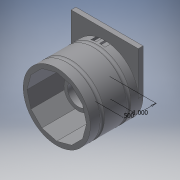
# Autodesk Inventor part: mounting plate
Saved by Autodesk Inventor 2017 (Build 210142000, 142)
## iProperties
Created: 2017-11-23
Part Number: mounting plate
Material: Generic
Document SubType Name: Modeling
Designer: prakh
Density: 1 g/cm^3
Appearance: Default
Author: prakh
Autodesk Inventor part; units mm, degrees
ref_plane "YZ Plane" through (0, 0, 0) normal (1, 0, 0) x (0, 1, 0)
ref_plane "XZ Plane" through (0, 0, 0) normal (0, 1, 0) x (-1, 0, 0)
ref_plane "XY Plane" through (0, 0, 0) normal (0, 0, 1) x (1, 0, 0)
sketch "Sketch1" plane through (0, 0, 0) normal (0, 0, 1) x (1, 0, 0)
  circle A0 centre (0, 0) radius 44.45
  line L0 (-44.45, 44.45) -> (44.45, 44.45)
  line L1 (44.45, 44.45) -> (44.45, -44.45)
  line L2 (44.45, -44.45) -> (-44.45, -44.45)
  line L3 (-44.45, -44.45) -> (-44.45, 44.45)
  dimension "d0" = 88.9
  dimension "d1" = 88.9
  dimension "d2" = 88.9
  dimension "d3" = 44.45
  dimension "d4" = 44.45
  constraints: 8 end point, 2 parallel, 1 centre point, 1 coincident, 1 horizontal, 1 perpendicular
  measures "d0" diameter of A0
  measures "d1" distance of L1.end L2.end
  measures "d2" distance of L0.end L1.end
  measures "d3" distance from line of point (0, 0) L1
  measures "d4" distance from line of point (0, 0) L0
extrude "Extrusion1" add sketch "Sketch1" along normal blind 6.35
sketch "Sketch2" plane through (0, 0, 6.35) normal (0, 0, 1) x (1, 0, 0)
  circle A0 centre (0, 0) radius 46.0375
  circle A1 centre (0, 0) radius 44.45
  line L0 (0, 39.444) -> (19.722, 34.1595)
  line L1 (19.722, 34.1595) -> (34.1595, 19.722)
  line L2 (34.1595, 19.722) -> (39.444, 0)
  line L3 (39.444, 0) -> (34.1595, -19.722)
  line L4 (34.1595, -19.722) -> (19.722, -34.1595)
  line L5 (19.722, -34.1595) -> (0, -39.444)
  line L6 (0, -39.444) -> (-19.722, -34.1595)
  line L7 (-19.722, -34.1595) -> (-34.1595, -19.722)
  line L8 (-34.1595, -19.722) -> (-39.444, 0)
  line L9 (-39.444, 0) -> (-34.1595, 19.722)
  line L10 (-34.1595, 19.722) -> (-19.722, 34.1595)
  line L11 (-19.722, 34.1595) -> (0, 39.444)
  dimension "d8" = 1.5875
  dimension "d25" = 76.2
  dimension "d46" = 88.9
  constraints: 24 end point, 3 coincident, 2 centre point, 25 other
  measures "d8" radial gap between concentric circles of A1 A0
  measures "d25" distance between parallel lines of L5 L11
  measures "d46" diameter of A1
extrude "Extrusion2" add sketch "Sketch2" along normal blind 63.5 contours A1
sketch "Sketch3" plane through (0, 0, 6.35) normal (0, 0, 1) x (1, 0, 0)
  circle A0 centre (0, 0) radius 14.2875
  dimension "d11" = 28.575
  constraints: 1 centre point, 1 coincident
  measures "d11" diameter of A0
extrude "Extrusion3" cut sketch "Sketch3" against normal blind 38.1
sketch "Sketch4" plane through (0, 0, 6.35) normal (0, 0, 1) x (1, 0, 0)
  circle A0 centre (0, 0) radius 14.2875 projected
  circle A1 centre (0, 0) radius 19.05
  dimension "d14" = 38.1
  constraints: 1 centre point, 1 coincident
  measures "d14" diameter of A1
extrude "Extrusion4" add sketch "Sketch4" along normal blind 34.925
sketch "Sketch6" plane through (0, 0, 6.35) normal (0, 0, 1) x (1, 0, 0)
  circle A0 centre (31.75, 0) radius 7.62
  point P0 (0, 0)
  dimension "d21" = 15.24
  dimension "d22" = 31.75
  constraints: 1 centre point, 1 horizontal alignment
  measures "d21" diameter of A0
  measures "d22" distance of point (0, 0) A0.centre
extrude "Extrusion6" cut sketch "Sketch6" against normal blind 25.4
sketch "Sketch7" plane through (0, 0, 6.35) normal (0, 0, 1) x (1, 0, 0)
  line L0 (0, 44.45) -> (-44.45, 44.45) projected
  line L1 (-44.45, 44.45) -> (-44.45, 0) projected
  line L2 (0, -44.45) -> (44.45, -44.45) projected
  line L3 (44.45, 0) -> (44.45, 44.45) projected
  arc A0 (44.45, 0) -> (0, 44.45) centre (0, 0) ccw projected
  line L4 (44.45, -44.45) -> (44.45, 44.45) projected
  arc A1 (0, 44.45) -> (-44.45, 0) centre (0, 0) ccw projected
  arc A2 (-44.45, 0) -> (0, -44.45) centre (0, 0) ccw projected
  line L5 (-44.45, 0) -> (-44.45, -44.45) projected
  line L6 (44.45, 44.45) -> (0, 44.45) projected
  arc A3 (0, -44.45) -> (44.45, 0) centre (0, 0) ccw projected
  line L7 (44.45, -44.45) -> (44.45, 0) projected
  line L8 (-44.45, -44.45) -> (0, -44.45) projected
  line L9 (-44.45, 0) -> (-44.45, -44.45)
  line L10 (-44.45, -44.45) -> (0, -44.45)
  line L11 (44.45, -44.45) -> (-44.45, -44.45) projected
  line L12 (0, -44.45) -> (44.45, -44.45)
  line L13 (44.45, -44.45) -> (44.45, 0)
  arc A4 (-44.45, 0) -> (0, -44.45) centre (0, 0) ccw
  arc A5 (0, -44.45) -> (44.45, 0) centre (0, 0) ccw
  point P0 (-44.4261, -1.4578)
  point P1 (44.4261, -1.4578)
  constraints: 8 end point, 4 point on circle, 2 centre point, 2 perpendicular, 2 tangent, 1 concentric, 1 horizontal, 1 vertical
extrude "Extrusion7" cut sketch "Sketch7" against normal blind 25.4 contours L4 L2 A3 | A2 L8 L5
sketch "Sketch8" plane through (0, 0, 0) normal (0, 1, 0) x (-1, 0, 0)
  line L0 (44.45, 0) -> (44.45, 69.85) projected
  arc A0 (44.45, 56.8325) -> (44.45, 51.1175) centre (45.974, 53.975) ccw
  arc A1 (44.45, 21.9075) -> (44.45, 16.1925) centre (45.974, 19.05) ccw
  line L1 (44.45, 69.85) -> (-44.45, 69.85) projected
  line L2 (0, -13.97) -> (0, 83.82) projected
  arc A2 (44.2147, 16.3311) -> (44.45, 21.9075) centre (45.974, 19.05) ccw
  point P0 (0, 0)
  dimension "d28" = 3.2385
  dimension "d31" = 19.05
  dimension "d32" = 15.875
  dimension "d45" = 1.7145
  constraints: 6 point on circle, 4 point on line, 3 centre point, 1 coincident, 1 equal radius, 1 vertical alignment
  measures "d28" radius of A1
  measures "d31" vertical distance of L0.start A1.centre
  measures "d32" distance from line of A0.centre L1
  measures "d45" distance edge to line of A1 L0
revolve "Revolution1" cut sketch "Sketch8" angle 360 about axis through (0, 0, -10) along (0, 0, 1) contours A1 L0 | A0 L0
sketch "Sketch9" plane through (0, 0, 6.35) normal (0, 0, 1) x (1, 0, 0)
  arc A0 (39.3642, -0.298) -> (39.3642, 0.298) centre (31.75, 0) ccw projected
  circle A1 centre (0, 0) radius 19.05 projected
  line L0 (34.1595, 19.722) -> (19.722, 34.1595) projected
  line L1 (19.722, 34.1595) -> (0, 39.444) projected
  line L2 (0, 39.444) -> (-19.722, 34.1595) projected
  line L3 (-19.722, 34.1595) -> (-34.1595, 19.722) projected
  line L4 (-34.1595, 19.722) -> (-39.444, 0) projected
  line L5 (-39.444, 0) -> (-34.1595, -19.722) projected
  line L6 (-34.1595, -19.722) -> (-19.722, -34.1595) projected
  line L7 (-19.722, -34.1595) -> (0, -39.444) projected
  line L8 (0, -39.444) -> (19.722, -34.1595) projected
  line L9 (19.722, -34.1595) -> (34.1595, -19.722) projected
  line L10 (34.1595, -19.722) -> (38.4931, -3.549) projected
  line L11 (39.444, 0) -> (39.3642, 0.298) projected
  circle A2 centre (0, -31.75) radius 4.826
  line L12 (39.3642, -0.298) -> (39.444, 0) projected
  arc A3 (38.4931, 3.549) -> (38.4931, -3.549) centre (31.75, 0) ccw projected
  line L13 (38.4931, 3.549) -> (34.1595, 19.722) projected
  dimension "d35" = 9.652
  dimension "d36" = 31.75
  dimension "d37" = 31.75
  constraints: 1 centre point, 1 vertical alignment
  measures "d35" diameter of A2
  measures "d36" distance of point (0, 0) A0.centre
  measures "d37" distance of A2.centre point (0, 0)
extrude "Extrusion8" cut sketch "Sketch9" against normal blind 25.4 contours A2
sketch "Sketch10" plane through (0, 0, 6.35) normal (0, 0, 1) x (1, 0, 0)
  circle A0 centre (0, -31.75) radius 4.826 projected
  arc A1 (39.3642, -0.298) -> (39.3642, 0.298) centre (31.75, 0) ccw projected
  circle A2 centre (0, 0) radius 19.05 projected
  line L0 (34.1595, 19.722) -> (19.722, 34.1595) projected
  line L1 (19.722, 34.1595) -> (0, 39.444) projected
  line L2 (0, 39.444) -> (-19.722, 34.1595) projected
  line L3 (-19.722, 34.1595) -> (-34.1595, 19.722) projected
  line L4 (-34.1595, 19.722) -> (-39.444, 0) projected
  line L5 (-39.444, 0) -> (-34.1595, -19.722) projected
  line L6 (-34.1595, -19.722) -> (-19.722, -34.1595) projected
  line L7 (-19.722, -34.1595) -> (0, -39.444) projected
  line L8 (0, -39.444) -> (19.722, -34.1595) projected
  line L9 (19.722, -34.1595) -> (34.1595, -19.722) projected
  line L10 (34.1595, -19.722) -> (38.4931, -3.549) projected
  line L11 (39.444, 0) -> (39.3642, 0.298) projected
  arc A3 (7.6781, -37.3867) -> (-7.6781, -37.3867) centre (0, -31.75) ccw
  line L12 (39.3642, -0.298) -> (39.444, 0) projected
  arc A4 (38.4931, 3.549) -> (38.4931, -3.549) centre (31.75, 0) ccw projected
  line L13 (38.4931, 3.549) -> (34.1595, 19.722) projected
  dimension "d40" = 19.05
  constraints: 2 point on circle, 2 point on line, 1 centre point, 1 coincident
  measures "d40" diameter of A3
extrude "Extrusion9" cut sketch "Sketch10" against normal blind 3.175 contours L8 L7 A3
sketch "Sketch11" plane through (0, 0, 0) normal (0, 1, 0) x (-1, 0, 0)
  line L0 (-19.05, 6.35) -> (-19.05, 41.275) projected
  line L1 (-19.05, 38.1) -> (-26.605, 25.4)
  line L2 (-26.605, 25.4) -> (-23.8011, 25.4)
  line L3 (44.45, 21.9075) -> (-44.45, 21.9075) projected
  line L4 (-23.8011, 25.4) -> (-17.684, 35.6829)
  point P0 (0, 0)
  dimension "d43" = 25.4
  dimension "d44" = 12.7
  constraints: 6 end point, 2 parallel, 1 point on line
  measures "d43" distance from line of point (0, 0) L2
  measures "d44" vertical distance of L1.start L1.end
sketch "Sketch12" plane through (-44.45, 44.45, 0) normal (0, 1, 0) x (1, 0, 0)
  line L0 (0, 0) -> (88.9, 0) projected
  line L1 (0, 0) -> (0, -6.35) projected
  line L2 (44.45, -6.35) -> (0, -6.35) projected
  line L3 (88.9, -6.35) -> (44.45, -6.35) projected
  line L4 (88.9, 0) -> (88.9, -6.35) projected
  point P0 (44.45, 0)
extrude "Extrusion10" add sketch "Sketch12" along normal blind 12.7
sketch "Sketch13" plane through (0, 0, 0) normal (0, 0, -1) x (-1, 0, 0)
  circle A0 centre (0, 0) radius 44.45 projected
  arc A1 (44.45, 0) -> (-44.45, 0) centre (0, 0) ccw projected
  line L0 (-7.4513, 43.821) -> (0.0223, 44.45)
  line L1 (0.0223, 44.45) -> (0.2739, 41.4606)
  line L2 (0.2739, 41.4606) -> (-7.1997, 40.8316)
  line L3 (-7.1997, 40.8316) -> (-7.4513, 43.821)
  line L4 (4.1443, 44.2564) -> (11.526, 42.9296)
  line L5 (11.526, 42.9296) -> (10.9953, 39.9769)
  line L6 (10.9953, 39.9769) -> (3.6136, 41.3037)
  line L7 (3.6136, 41.3037) -> (4.1443, 44.2564)
  line L8 (0, 0) -> (0, 64.8467) construction
  line L9 (0, 0) -> (-11.2605, 63.8615) construction
  line L10 (0, 0) -> (-22.1789, 60.936) construction
  line L11 (0, 0) -> (-32.4234, 56.1589) construction
  line L12 (0, 0) -> (-41.6827, 49.6755) construction
  line L13 (0, 0) -> (-49.6755, 41.6827) construction
  line L14 (0, 0) -> (-56.1589, 32.4234) construction
  line L15 (0, 0) -> (-60.936, 22.1789) construction
  line L16 (0, 0) -> (-63.8615, 11.2605) construction
  line L17 (0, 0) -> (-64.8467, 0) construction
  line L18 (0, 0) -> (-63.8615, -11.2605) construction
  line L19 (0, 0) -> (-60.936, -22.1789) construction
  line L20 (0, 0) -> (-56.1589, -32.4234) construction
  line L21 (0, 0) -> (-49.6755, -41.6827) construction
  line L22 (0, 0) -> (-41.6827, -49.6755) construction
  line L23 (0, 0) -> (-32.4234, -56.1589) construction
  line L24 (0, 0) -> (-22.1789, -60.936) construction
  line L25 (0, 0) -> (-11.2605, -63.8615) construction
  line L26 (0, 0) -> (0, -64.8467) construction
  line L27 (0, 0) -> (11.2605, -63.8615) construction
  line L28 (0, 0) -> (22.1789, -60.936) construction
  line L29 (0, 0) -> (32.4234, -56.1589) construction
  line L30 (0, 0) -> (41.6827, -49.6755) construction
  line L31 (0, 0) -> (49.6755, -41.6827) construction
  line L32 (0, 0) -> (56.1589, -32.4234) construction
  line L33 (0, 0) -> (60.936, -22.1789) construction
  line L34 (0, 0) -> (63.8615, -11.2605) construction
  line L35 (0, 0) -> (64.8467, 0) construction
  line L36 (0, 0) -> (63.8615, 11.2605) construction
  line L37 (0, 0) -> (60.936, 22.1789) construction
  line L38 (0, 0) -> (56.1589, 32.4234) construction
  line L39 (0, 0) -> (49.6755, 41.6827) construction
  line L40 (0, 0) -> (41.6827, 49.6755) construction
  line L41 (0, 0) -> (32.4234, 56.1589) construction
  line L42 (0, 0) -> (22.1789, 60.936) construction
  line L43 (0, 0) -> (11.2605, 63.8615) construction
  point P0 (0, -44.45)
  dimension "d53" = 7.5
  dimension "d54" = 3
  dimension "d55" = 3
  dimension "d56" = 7.5
  dimension "d59" = 360
  dimension "d61" = 15
  constraints: 88 end point, 4 parallel, 4 point on circle, 2 perpendicular, 1 point on line, 1 vertical, 114 other
  measures "d53" distance of L4.start L4.end
  measures "d54" distance of L4.end L5.end
  measures "d55" distance of L0.end L1.end
  measures "d56" distance of L0.start L0.end
  measures "d61" angle of L7 L1
extrude "Extrusion11" cut sketch "Sketch13" against normal blind 13.35 contours L4 A0 | L5 L6 L7 L4 | A0 L0 | L0 L1 L2 L3
sketch "Sketch14" plane through (0, 0, 0) normal (0, 0, -1) x (-1, 0, 0)
  circle A0 centre (10.2313, 30.0563) radius 2.4575
  circle A1 centre (-15.0804, 27.94) radius 2.4575
  circle A2 centre (-22.5999, -22.3004) radius 2.4575
  circle A3 centre (0, 0) radius 14.2875 projected
  dimension "d64" = 4.9149
  dimension "d71" = 31.75
  dimension "d72" = 31.75
  dimension "d73" = 31.75
  dimension "d74" = 25.4
  dimension "d75" = 50.8
  dimension "d76" = 27.94
  constraints: 3 centre point, 2 equal radius
  measures "d64" diameter of A1
  measures "d71" distance of A3.centre A2.centre
  measures "d72" distance of A1.centre point (0, 0)
  measures "d73" distance of A0.centre point (0, 0)
  measures "d74" distance of A0.centre A1.centre
  measures "d75" distance of A2.centre A1.centre
  measures "d76" vertical distance of A1.centre point (0, 0)
extrude "Extrusion12" cut sketch "Sketch14" against normal blind 25.4 contours A0 | A1 | A2
equation "\"d3\" = 0.5 * d1"
equation "\"d4\" = 0.5 * d2"
equation "\"d37\" = d36"
equation "\"d55\" = d54"
equation "\"d56\" = d53"
body "Solid1"
